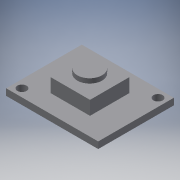
# Autodesk Inventor part: optical
Saved by Autodesk Inventor 2019 (Build 230136000, 136)
## iProperties
Created: 2020-03-22
Part Number: optical
Material: Generic
Document SubType Name: Modeling
Designer: Pulag
Density: 1 g/cm^3
Appearance: Default
Author: Pulag
Autodesk Inventor part; units mm, degrees
ref_plane "YZ Plane" through (0, 0, 0) normal (1, 0, 0) x (0, 1, 0)
ref_plane "XZ Plane" through (0, 0, 0) normal (0, 1, 0) x (-1, 0, 0)
ref_plane "XY Plane" through (0, 0, 0) normal (0, 0, 1) x (1, 0, 0)
sketch "Sketch1" plane through (0, 0, 0) normal (0, 1, 0) x (-1, 0, 0)
  line L0 (-7, 5.75) -> (7, 5.75)
  line L1 (7, 5.75) -> (7, -5.75)
  line L2 (7, -5.75) -> (-7, -5.75)
  line L3 (-7, -5.75) -> (-7, 5.75)
  line L4 (7, 5.75) -> (-7, -5.75) construction
  line L5 (-7, -5.75) -> (-5.8, -5.75)
  line L6 (-7, -4.55) -> (-7, -5.75)
  line L7 (7, 5.75) -> (5.8, 5.75)
  line L8 (7, 4.55) -> (7, 5.75)
  circle A0 centre (-5.8, -4.55) radius 0.7
  circle A1 centre (5.8, 4.55) radius 0.7
  line L9 (-3, 3) -> (3, 3)
  line L10 (3, 3) -> (3, -3)
  line L11 (3, -3) -> (-3, -3)
  line L12 (-3, -3) -> (-3, 3)
  line L13 (-3, 3) -> (3, -3) construction
  line L14 (3, 3) -> (-3, -3) construction
  circle A2 centre (0.5, -0.45) radius 1.885
  point P0 (3.3, -2.75)
  point P1 (0, 0)
  dimension "d0" = 14
  dimension "d1" = 11.5
  dimension "d6" = 1.4
  dimension "d7" = 1.4
  dimension "d12" = 6
  dimension "d13" = 6
  dimension "d17" = 3.77
  constraints: 30 end point, 4 horizontal, 4 parallel, 3 centre point, 3 midpoint, 2 perpendicular
  measures "d0" distance of L1.end L2.end
  measures "d1" distance of L0.end L1.end
  measures "d6" diameter of A0
  measures "d7" diameter of A1
  measures "d12" distance of L10.end L11.end
  measures "d13" distance of L9.end L10.end
  measures "d17" diameter of A2
sketch "Sketch2" plane through (0, 0, 0) normal (0, 1, 0) x (-1, 0, 0)
  line L0 (-7, 5.75) -> (7, 5.75)
  line L1 (7, 5.75) -> (7, -5.75)
  line L2 (7, -5.75) -> (-7, -5.75)
  line L3 (-7, -5.75) -> (-7, 5.75)
  line L4 (7, 5.75) -> (-7, -5.75) construction
  line L5 (-7, -5.75) -> (-5.8, -5.75)
  line L6 (-7, -4.55) -> (-7, -5.75)
  line L7 (7, 5.75) -> (5.8, 5.75)
  line L8 (7, 4.55) -> (7, 5.75)
  circle A0 centre (-5.8, -4.55) radius 0.7
  circle A1 centre (5.8, 4.55) radius 0.7
  line L9 (-3, 3) -> (3, 3)
  line L10 (3, 3) -> (3, -3)
  line L11 (3, -3) -> (-3, -3)
  line L12 (-3, -3) -> (-3, 3)
  line L13 (-3, 3) -> (3, -3) construction
  line L14 (3, 3) -> (-3, -3) construction
  circle A2 centre (0.5, -0.45) radius 1.885
  point P0 (0, 0)
  point P1 (3.3, -2.75)
  point P2 (0, 0)
  dimension "d18" = 14
  dimension "d19" = 11.5
  dimension "d20" = 1.4
  dimension "d21" = 1.4
  dimension "d22" = 6
  dimension "d23" = 6
  dimension "d24" = 3.77
  constraints: 30 end point, 4 horizontal, 4 parallel, 3 centre point, 3 midpoint, 2 perpendicular
  measures "d18" distance of L1.end L2.end
  measures "d19" distance of L0.end L1.end
  measures "d20" diameter of A0
  measures "d21" diameter of A1
  measures "d22" distance of L10.end L11.end
  measures "d23" distance of L9.end L10.end
  measures "d24" diameter of A2
sketch "Sketch3" plane through (0, 0, 0) normal (0, 1, 0) x (-1, 0, 0)
  line L0 (-7, 5.75) -> (7, 5.75)
  line L1 (7, 5.75) -> (7, -5.75)
  line L2 (7, -5.75) -> (-7, -5.75)
  line L3 (-7, -5.75) -> (-7, 5.75)
  line L4 (7, 5.75) -> (-7, -5.75) construction
  line L5 (-7, -5.75) -> (-5.8, -5.75)
  line L6 (-7, -4.55) -> (-7, -5.75)
  line L7 (7, 5.75) -> (5.8, 5.75)
  line L8 (7, 4.55) -> (7, 5.75)
  circle A0 centre (-5.8, -4.55) radius 0.7
  circle A1 centre (5.8, 4.55) radius 0.7
  line L9 (-3, 3) -> (3, 3)
  line L10 (3, 3) -> (3, -3)
  line L11 (3, -3) -> (-3, -3)
  line L12 (-3, -3) -> (-3, 3)
  line L13 (-3, 3) -> (3, -3) construction
  line L14 (3, 3) -> (-3, -3) construction
  circle A2 centre (0.5, -0.45) radius 1.885
  point P0 (0, 0)
  point P1 (3.3, -2.75)
  point P2 (0, 0)
  dimension "d25" = 14
  dimension "d26" = 11.5
  dimension "d27" = 1.4
  dimension "d28" = 1.4
  dimension "d29" = 6
  dimension "d30" = 6
  dimension "d31" = 3.77
  constraints: 30 end point, 4 horizontal, 4 parallel, 3 centre point, 3 midpoint, 2 perpendicular
  measures "d25" distance of L1.end L2.end
  measures "d26" distance of L0.end L1.end
  measures "d27" diameter of A0
  measures "d28" diameter of A1
  measures "d29" distance of L10.end L11.end
  measures "d30" distance of L9.end L10.end
  measures "d31" diameter of A2
extrude "Extrusion1" add sketch "Sketch1" against normal blind 1 contours L0 L1 L2 L3 | L9 L10 L11 L12 | A2
extrude "Extrusion2" add sketch "Sketch2" along normal blind 2.1 contours L9 L10 L11 L12 | A2
extrude "Extrusion3" add sketch "Sketch3" along normal blind 0.7 from surface at 2.1 contours A2
sketch "Sketch4" plane through (0, -1, 0) normal (0, -1, 0) x (1, 0, 0)
  line L0 (3, -3) -> (-3, -3)
  line L1 (-3, -3) -> (-3, 3)
  line L2 (-3, 3) -> (3, 3)
  line L3 (3, 3) -> (3, -3)
  line L4 (3, -3) -> (-3, 3) construction
  line L5 (-3, -3) -> (3, 3) construction
  point P0 (0, 0)
  dimension "d38" = 6
  dimension "d39" = 6
  constraints: 12 end point, 2 midpoint, 2 parallel, 1 horizontal, 1 perpendicular
  measures "d38" distance of L1.end L2.end
  measures "d39" distance of L0.end L1.end
extrude "Extrusion4" add sketch "Sketch4" along normal blind 1
body "Solid1"
